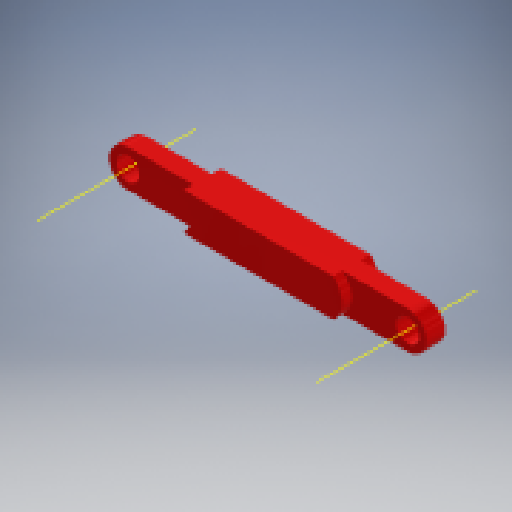
# Autodesk Inventor part: link7
Saved by Autodesk Inventor 2024.1 (Build 281209000, 209)
## iProperties
Created: 2023-09-09
Part Number: link7
Material: Aluminum 6061
Document SubType Name: Modeling
Designer: Camilo
Density: 2.7 g/cm^3
Appearance: Aluminum - Flat
Mass: 1.05543 g
Surface Area: 5.12076 cm^2
Volume: 0.390898 cm^3
Author: Camilo
Autodesk Inventor part; units mm, degrees
ref_plane "YZ Plane" through (0, 0, 0) normal (1, 0, 0) x (0, 1, 0)
ref_plane "XZ Plane" through (0, 0, 0) normal (0, 1, 0) x (-1, 0, 0)
ref_plane "XY Plane" through (0, 0, 0) normal (0, 0, 1) x (1, 0, 0)
sketch "Sketch1" plane through (0, 0, 0) normal (0, 0, 1) x (1, 0, 0)
  line L0 (0, 0) -> (15, 0)
  line L1 (0, 0) -> (-15, 0)
  line L2 (0, 0) -> (5, 0)
  circle A0 centre (-15, 0) radius 1.25
  circle A1 centre (15, 0) radius 1.25
  circle A2 centre (-15, 0) radius 2
  circle A3 centre (15, 0) radius 2
  line L3 (-15, 2) -> (15, 2)
  line L4 (-15, -2) -> (15, -2)
  line L5 (-15, 2) -> (-8, 2)
  line L6 (-8, 2) -> (-8, -2)
  line L7 (-8, -2) -> (-15, -2)
  line L8 (-15, -2) -> (-15, 2)
  line L9 (15, 2) -> (12.5, 2)
  line L10 (15, -2) -> (15, 2)
  arc A4 (-8, -2) -> (-8, 2) centre (-10.2361, 0) ccw
  line L11 (5, 0) -> (1, 0)
  line L12 (5, 2) -> (5, 2)
  line L13 (5, 0) -> (9, 0)
  line L14 (-15, 2) -> (-14.5, 2)
  line L15 (-15, -2) -> (-14.5, -2)
  arc A5 (-14.5, -2) -> (-14.5, 2) centre (-14.5, 0) ccw
  line L16 (15, 0) -> (7, 0)
  line L17 (15, 2) -> (5, 2)
  line L18 (15, -2) -> (5, -2)
  arc A6 (5, -2) -> (5, 2) centre (5, 0) ccw
  point P0 (-8, 2)
  dimension "d1" = 15
  dimension "d2" = 15
  dimension "d4" = 2.5
  dimension "d6" = 2.5
  dimension "d7" = 4
  dimension "d8" = 4
  dimension "d10" = 7
  dimension "d16" = 4
  dimension "d17" = 3
  dimension "d24" = 0.5
  dimension "d25" = 0.5
  dimension "d26" = 2
  dimension "d37" = 8
  dimension "d44" = 10
  dimension "d45" = 10
  constraints: 38 end point, 11 point on circle, 10 point on line, 7 centre point, 5 coincident, 4 horizontal, 2 parallel, 2 tangent, 1 collinear, 1 perpendicular
  measures "d1" distance of L0.start L0.end
  measures "d2" distance of L0.start L1.end
  measures "d4" diameter of A0
  measures "d6" diameter of A1
  measures "d7" diameter of A2
  measures "d8" diameter of A3
  measures "d10" distance of L6.end L7.end
  measures "d16" distance of L3.start L4.start
  measures "d17" radius of A4
  measures "d24" distance of L3.start L14.end
  measures "d25" distance of L7.end L15.end
  measures "d26" radius of A5
  measures "d37" distance of L16.start L16.end
  measures "d44" distance from line of L12.end L10
  measures "d45" distance from line of L18.end L10
extrude "Extrusion6" add sketch "Sketch1" along normal mid plane 2 contours A4 L6 L1 | L1 L6 A4 | L6 L4 A5 L1 | L1 A5 L3 L6 | A6 L3 A3 L0 | L0 A3 L4 A6 | A5 L4 A2 L1 | L1 A2 L3 A5 | A2 L8 A0 L1 | L1 A0 L8 A2 | A2 L8 A0 | L10 A1 A3 | A3 L0 A1 L10 | A3 L10 A1 L0
extrude "Extrusion7" add sketch "Sketch1" along normal mid plane 4 contours L1 A4 L3 A6 L0 | L0 A6 L4 A4 L1
body "Solid2"
